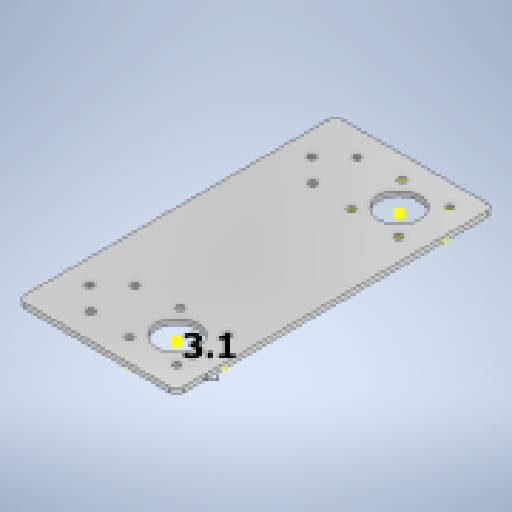
# Autodesk Inventor part: body_bottom_frame
Saved by Autodesk Inventor 2025.2 (Build 292293000, 293)
## iProperties
Created: 2025-08-01
Part Number: body_bottom_frame
Material: Aluminum 6061-AHC
Document SubType Name: Sheet Metal
Designer: chris
Density: 2.7 g/cm^3
Sheet Metal Rule: Default_mm
Appearance: Aluminum - Dark
Author: chris
Autodesk Inventor part; units mm, degrees
ref_plane "YZ Plane" through (0, 0, 0) normal (1, 0, 0) x (0, 1, 0)
ref_plane "XZ Plane" through (0, 0, 0) normal (0, 1, 0) x (-1, 0, 0)
ref_plane "XY Plane" through (0, 0, 0) normal (0, 0, 1) x (1, 0, 0)
sketch "Sketch1" plane through (0, 0, 0) normal (0, 1, 0) x (-1, 0, 0)
  line L0 (-30, 55) -> (30, 55)
  line L1 (30, 55) -> (30, -55)
  line L2 (30, -55) -> (-30, -55)
  line L3 (-30, -55) -> (-30, 55)
  line L4 (-30, 55) -> (30, -55) construction
  line L5 (30, 55) -> (-30, -55) construction
  point P0 (0, 0)
  dimension "d0" = 60
  dimension "d1" = 110
  measures "d0" distance of L1.end L2.end
  measures "d1" distance of L0.end L1.end
extrude "Plate1" add sketch "Sketch1" along normal blind 1.5
fillet "Fillet1" radius 2 4 edges at (30, 0.75, 55) (30, 0.75, -55) (-30, 0.75, -55) (-30, 0.75, 55)
sketch "Sketch5" plane through (0, 1.5, 0) normal (0, 1, 0) x (1, 0, 0)
  circle A0 centre (-17.42, -34.93) radius 0.7835 projected
  circle A1 centre (-10.12, -41.93) radius 0.7835 projected
  circle A2 centre (-10.12, -27.93) radius 0.7835 projected
  circle A3 centre (3.1, -42.93) radius 0.7835 projected
  circle A4 centre (3.1, -26.93) radius 0.7835 projected
  line L0 (-18.82, -28.86) -> (-18.82, -41) projected
  line L1 (-18.82, -28.86) -> (-18.1, -28.86) projected
  arc A5 (-18.1, -28.86) -> (-16.1, -26.86) centre (-18.1, -26.86) ccw projected
  line L2 (-16.1, -26.86) -> (-16.1, -26.14) projected
  line L3 (16, -26.14) -> (-16.1, -26.14) projected
  line L4 (16, -26.14) -> (16, -26.86) projected
  arc A6 (16, -26.86) -> (18, -28.86) centre (18, -26.86) ccw projected
  line L5 (18, -28.86) -> (18.72, -28.86) projected
  line L6 (18.72, -41) -> (18.72, -28.86) projected
  line L7 (18.72, -41) -> (18, -41) projected
  arc A7 (18, -41) -> (16, -43) centre (18, -43) ccw projected
  line L8 (16, -43) -> (16, -43.72) projected
  line L9 (-16.1, -43.72) -> (16, -43.72) projected
  line L10 (-16.1, -43.72) -> (-16.1, -43) projected
  arc A8 (-16.1, -43) -> (-18.1, -41) centre (-18.1, -43) ccw projected
  line L11 (-18.1, -41) -> (-18.82, -41) projected
  circle A9 centre (10, -34.93) radius 6.4 projected
  circle A10 centre (-17.42, 34.93) radius 0.7835 projected
  circle A11 centre (-10.12, 27.93) radius 0.7835 projected
  circle A12 centre (-10.12, 41.93) radius 0.7835 projected
  circle A13 centre (3.1, 26.93) radius 0.7835 projected
  circle A14 centre (3.1, 42.93) radius 0.7835 projected
  line L12 (-18.82, 41) -> (-18.82, 28.86) projected
  line L13 (-18.82, 41) -> (-18.1, 41) projected
  arc A15 (-18.1, 41) -> (-16.1, 43) centre (-18.1, 43) ccw projected
  line L14 (-16.1, 43) -> (-16.1, 43.72) projected
  line L15 (16, 43.72) -> (-16.1, 43.72) projected
  line L16 (16, 43.72) -> (16, 43) projected
  arc A16 (16, 43) -> (18, 41) centre (18, 43) ccw projected
  line L17 (18, 41) -> (18.72, 41) projected
  line L18 (18.72, 28.86) -> (18.72, 41) projected
  line L19 (18.72, 28.86) -> (18, 28.86) projected
  arc A17 (18, 28.86) -> (16, 26.86) centre (18, 26.86) ccw projected
  line L20 (16, 26.86) -> (16, 26.14) projected
  line L21 (-16.1, 26.14) -> (16, 26.14) projected
  line L22 (-16.1, 26.14) -> (-16.1, 26.86) projected
  arc A18 (-16.1, 26.86) -> (-18.1, 28.86) centre (-18.1, 26.86) ccw projected
  line L23 (-18.1, 28.86) -> (-18.82, 28.86) projected
  circle A19 centre (10, 34.93) radius 6.4 projected
  point P0 (0, 0)
hole "Hole3" at (-17.42, 1.5, 34.93) at (-10.12, 1.5, 27.93) at (-10.12, 1.5, 41.93) at (3.1, 1.5, 42.93) at (3.1, 1.5, 26.93) at (18, 1.5, 26.86) at (18, 1.5, 43) at (18, 1.5, -26.86) at (18, 1.5, -43) at (3.1, 1.5, -42.93) at (3.1, 1.5, -26.93) at (-10.12, 1.5, -41.93) at (-10.12, 1.5, -27.93) at (-17.42, 1.5, -34.93) direction (0, -1, 0) diameter 2.1 depth 1.5 tip angle 118
sketch "Sketch6" plane through (0, 1.5, 0) normal (0, 1, 0) x (1, 0, 0)
  circle A0 centre (-17.42, -34.93) radius 0.7835 projected
  circle A1 centre (-10.12, -41.93) radius 0.7835 projected
  circle A2 centre (-10.12, -27.93) radius 0.7835 projected
  circle A3 centre (3.1, -42.93) radius 0.7835 projected
  circle A4 centre (3.1, -26.93) radius 0.7835 projected
  line L0 (-18.82, -28.86) -> (-18.82, -41) projected
  line L1 (-18.82, -28.86) -> (-18.1, -28.86) projected
  arc A5 (-18.1, -28.86) -> (-16.1, -26.86) centre (-18.1, -26.86) ccw projected
  line L2 (-16.1, -26.86) -> (-16.1, -26.14) projected
  line L3 (16, -26.14) -> (-16.1, -26.14) projected
  line L4 (16, -26.14) -> (16, -26.86) projected
  arc A6 (16, -26.86) -> (18, -28.86) centre (18, -26.86) ccw projected
  line L5 (18, -28.86) -> (18.72, -28.86) projected
  line L6 (18.72, -41) -> (18.72, -28.86) projected
  line L7 (18.72, -41) -> (18, -41) projected
  arc A7 (18, -41) -> (16, -43) centre (18, -43) ccw projected
  line L8 (16, -43) -> (16, -43.72) projected
  line L9 (-16.1, -43.72) -> (16, -43.72) projected
  line L10 (-16.1, -43.72) -> (-16.1, -43) projected
  arc A8 (-16.1, -43) -> (-18.1, -41) centre (-18.1, -43) ccw projected
  line L11 (-18.1, -41) -> (-18.82, -41) projected
  circle A9 centre (10, -34.93) radius 6.4 projected
  circle A10 centre (-17.42, 34.93) radius 0.7835 projected
  circle A11 centre (-10.12, 27.93) radius 0.7835 projected
  circle A12 centre (-10.12, 41.93) radius 0.7835 projected
  circle A13 centre (3.1, 26.93) radius 0.7835 projected
  circle A14 centre (3.1, 42.93) radius 0.7835 projected
  line L12 (-18.82, 41) -> (-18.82, 28.86) projected
  line L13 (-18.82, 41) -> (-18.1, 41) projected
  arc A15 (-18.1, 41) -> (-16.1, 43) centre (-18.1, 43) ccw projected
  line L14 (-16.1, 43) -> (-16.1, 43.72) projected
  line L15 (16, 43.72) -> (-16.1, 43.72) projected
  line L16 (16, 43.72) -> (16, 43) projected
  arc A16 (16, 43) -> (18, 41) centre (18, 43) ccw projected
  line L17 (18, 41) -> (18.72, 41) projected
  line L18 (18.72, 28.86) -> (18.72, 41) projected
  line L19 (18.72, 28.86) -> (18, 28.86) projected
  arc A17 (18, 28.86) -> (16, 26.86) centre (18, 26.86) ccw projected
  line L20 (16, 26.86) -> (16, 26.14) projected
  line L21 (-16.1, 26.14) -> (16, 26.14) projected
  line L22 (-16.1, 26.14) -> (-16.1, 26.86) projected
  arc A18 (-16.1, 26.86) -> (-18.1, 28.86) centre (-18.1, 26.86) ccw projected
  line L23 (-18.1, 28.86) -> (-18.82, 28.86) projected
  circle A19 centre (10, 34.93) radius 6.4 projected
  circle A20 centre (10, -34.93) radius 6.5
  circle A21 centre (10, 34.93) radius 6.5
  point P0 (0, 0)
  dimension "d27" = 13
  dimension "d28" = 13
  constraints: 2 centre point, 2 coincident
  measures "d27" diameter of A20
  measures "d28" diameter of A21
extrude "Cut2" cut sketch "Sketch6" against normal blind 1.5 contours A9 | A19 | A20 | A21
sketch "Sketch8" plane through (0, 0, 0) normal (0, -1, 0) x (1, 0, 0)
  circle A0 centre (10, 34.93) radius 20 projected
  arc A1 (1.8062, 40.9373) -> (1.7565, 41.5865) centre (1.403, 41.2329) ccw projected
  arc A2 (4.6263, 44.0616) -> (1.7565, 41.5865) centre (3.1, 42.93) ccw projected
  arc A3 (4.6263, 44.0616) -> (5.2611, 43.9171) centre (5.0279, 44.3594) ccw projected
  arc A4 (15.5012, 43.4718) -> (5.2611, 43.9171) centre (10, 34.93) ccw projected
  arc A5 (15.5012, 43.4718) -> (16.2361, 43.7063) centre (15.772, 43.8921) ccw projected
  arc A6 (18.7216, 41.2424) -> (16.2361, 43.7063) centre (18, 43) ccw projected
  arc A7 (18.7216, 41.2424) -> (18.4935, 40.5054) centre (18.9115, 40.7798) ccw projected
  arc A8 (18.4935, 29.3546) -> (18.4935, 40.5054) centre (10, 34.93) ccw projected
  arc A9 (18.4935, 29.3546) -> (18.7216, 28.6176) centre (18.9115, 29.0802) ccw projected
  arc A10 (16.2361, 26.1537) -> (18.7216, 28.6176) centre (18, 26.86) ccw projected
  arc A11 (16.2361, 26.1537) -> (15.5012, 26.3882) centre (15.772, 25.9679) ccw projected
  arc A12 (5.2611, 25.9429) -> (15.5012, 26.3882) centre (10, 34.93) ccw projected
  arc A13 (5.2611, 25.9429) -> (4.6263, 25.7984) centre (5.0279, 25.5006) ccw projected
  arc A14 (1.7565, 28.2735) -> (4.6263, 25.7984) centre (3.1, 26.93) ccw projected
  arc A15 (1.7565, 28.2735) -> (1.8062, 28.9227) centre (1.403, 28.6271) ccw projected
  arc A16 (1.8062, 40.9373) -> (1.8062, 28.9227) centre (10, 34.93) ccw projected
  circle A17 centre (10, -34.93) radius 20 projected
  arc A18 (1.8062, -28.9227) -> (1.7565, -28.2735) centre (1.403, -28.6271) ccw projected
  arc A19 (4.6263, -25.7984) -> (1.7565, -28.2735) centre (3.1, -26.93) ccw projected
  arc A20 (4.6263, -25.7984) -> (5.2611, -25.9429) centre (5.0279, -25.5006) ccw projected
  arc A21 (15.5012, -26.3882) -> (5.2611, -25.9429) centre (10, -34.93) ccw projected
  arc A22 (15.5012, -26.3882) -> (16.2361, -26.1537) centre (15.772, -25.9679) ccw projected
  arc A23 (18.7216, -28.6176) -> (16.2361, -26.1537) centre (18, -26.86) ccw projected
  arc A24 (18.7216, -28.6176) -> (18.4935, -29.3546) centre (18.9115, -29.0802) ccw projected
  arc A25 (18.4935, -40.5054) -> (18.4935, -29.3546) centre (10, -34.93) ccw projected
  arc A26 (18.4935, -40.5054) -> (18.7216, -41.2424) centre (18.9115, -40.7798) ccw projected
  arc A27 (16.2361, -43.7063) -> (18.7216, -41.2424) centre (18, -43) ccw projected
  arc A28 (16.2361, -43.7063) -> (15.5012, -43.4718) centre (15.772, -43.8921) ccw projected
  arc A29 (5.2611, -43.9171) -> (15.5012, -43.4718) centre (10, -34.93) ccw projected
  arc A30 (5.2611, -43.9171) -> (4.6263, -44.0616) centre (5.0279, -44.3594) ccw projected
  arc A31 (1.7565, -41.5865) -> (4.6263, -44.0616) centre (3.1, -42.93) ccw projected
  arc A32 (1.7565, -41.5865) -> (1.8062, -40.9373) centre (1.403, -41.2329) ccw projected
  arc A33 (1.8062, -28.9227) -> (1.8062, -40.9373) centre (10, -34.93) ccw projected
  line L0 (20, 25.86) -> (20, 44) projected
  line L1 (19, 24.86) -> (-19.1, 24.86) projected
  line L2 (-19.1, 45) -> (19, 45) projected
  line L3 (-19.1, -24.86) -> (19, -24.86) projected
  line L4 (20, -44) -> (20, -25.86) projected
  line L5 (19, -45) -> (-19.1, -45) projected
  circle A34 centre (25, 34.93) radius 2.8
  circle A35 centre (10, 49.93) radius 2.8
  circle A36 centre (10, 19.93) radius 2.8
  circle A37 centre (25, -34.93) radius 2.8
  circle A38 centre (10, -19.93) radius 2.8
  circle A39 centre (10, -49.93) radius 2.8
  line L6 (30, 53) -> (30, -53) projected
  line L7 (-28, 55) -> (28, 55) projected
  line L8 (28, -55) -> (-28, -55) projected
  point P0 (0, 0)
  dimension "d32" = 5.6
  dimension "d33" = 5.6
  dimension "d34" = 5.6
  dimension "d35" = 5.6
  dimension "d36" = 5.6
  dimension "d37" = 5.6
  dimension "d38" = 15
  dimension "d39" = 15
  dimension "d40" = 15
  dimension "d41" = 15
  dimension "d42" = 15
  dimension "d43" = 15
  dimension "d44" = 20
  dimension "d45" = 20
  dimension "d46" = 20
  dimension "d47" = 20
  dimension "d48" = 20.07
  dimension "d49" = 20.07
  constraints: 6 centre point
  measures "d32" diameter of A34
  measures "d33" diameter of A35
  measures "d34" diameter of A36
  measures "d35" diameter of A37
  measures "d36" diameter of A38
  measures "d37" diameter of A39
  measures "d38" distance of A35.centre A0.centre
  measures "d39" distance of A0.centre A36.centre
  measures "d40" distance of A0.centre A34.centre
  measures "d41" distance of A38.centre A17.centre
  measures "d42" distance of A39.centre A17.centre
  measures "d43" distance of A37.centre A17.centre
  measures "d44" distance from line of A36.centre L6
  measures "d45" distance from line of L6 A35.centre
  measures "d46" distance from line of L6 A38.centre
  measures "d47" distance from line of L6 A39.centre
  measures "d48" distance from line of A34.centre L7
  measures "d49" distance from line of L8 A37.centre
hole "Hole4" at (10, 0, 49.93) at (25, 0, 34.93) at (10, 0, 19.93) at (10, 0, -19.93) at (25, 0, -34.93) at (10, 0, -49.93) direction (0, 1, 0) diameter 3.1 depth 1.5 tip angle 118
equation "\"d25\" = Thickness"
equation "\"d29\" = Thickness"
equation "\"d2\" = Thickness"
equation "\"BendReliefWidth\" = Thickness"
equation "\"BendReliefDepth\" = 0.5 * Thickness"
equation "\"CornerReliefSize\" = 4 * Thickness"
equation "\"MinimumRemnant\" = 2 * Thickness"
equation "\"TransitionRadius\" = BendRadius"
equation "\"JacobiRadiusSize\" = BendRadius"
equation "\"GapSize\" = Thickness"
equation "\"Thickness\" = 1.5"
equation "\"BendRadius\" = 0.31"
body "Solid1"
